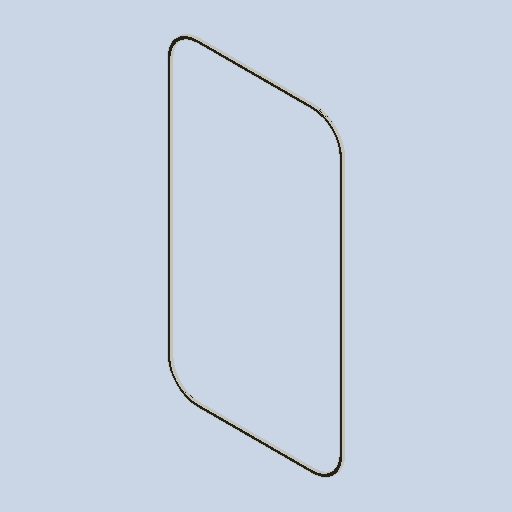
# Autodesk Inventor part: Caucho
Saved by Autodesk Inventor 2022.4 (Build 264492000, 492)
## iProperties
Created: 2022-11-28
Part Number: Caucho
Material: Generic
Document SubType Name: Sheet Metal
Designer: David
Density: 1 g/cm^3
Sheet Metal Rule: Default
Appearance: Gunmetal
Author: David
Autodesk Inventor part; units mm, degrees
ref_plane "YZ Plane" through (0, 0, 0) normal (1, 0, 0) x (0, 1, 0)
ref_plane "XZ Plane" through (0, 0, 0) normal (0, 1, 0) x (-1, 0, 0)
ref_plane "XY Plane" through (0, 0, 0) normal (0, 0, 1) x (1, 0, 0)
sketch "Sketch5" plane through (0, 0, 0) normal (0, 0, 1) x (1, 0, 0)
  line L0 (-300, -1100) -> (900, -1100)
  line L1 (900, -1100) -> (900, 850)
  line L2 (900, 850) -> (-300, 850)
  line L3 (-300, 850) -> (-300, -1100)
  line L4 (-300, -1100) -> (900, 850) construction
  line L5 (900, -1100) -> (-300, 850) construction
  line L6 (0, 700) -> (600, 700)
  line L7 (750, 550) -> (750, -800)
  line L8 (600, -950) -> (0, -950)
  line L9 (-150, -800) -> (-150, 550)
  arc A0 (750, 550) -> (600, 700) centre (600, 550) ccw
  arc A1 (0, 700) -> (-150, 550) centre (0, 550) ccw
  arc A2 (-150, -800) -> (0, -950) centre (0, -800) ccw
  arc A3 (600, -950) -> (750, -800) centre (600, -800) ccw
  line L10 (600, 697) -> (0, 697)
  arc A4 (0, 697) -> (-147, 550) centre (0, 550) ccw
  line L11 (-147, 550) -> (-147, -800)
  arc A5 (-147, -800) -> (0, -947) centre (0, -800) ccw
  line L12 (0, -947) -> (600, -947)
  arc A6 (600, -947) -> (747, -800) centre (600, -800) ccw
  line L13 (747, -800) -> (747, 550)
  arc A7 (747, 550) -> (600, 697) centre (600, 550) ccw
  point P0 (0, 0)
  point P1 (300, -125)
  dimension "d0" = 1200
  dimension "d1" = 1950
  dimension "d2" = 150
  dimension "d3" = 150
  dimension "d4" = 150
  dimension "d5" = 150
  dimension "d6" = 150
  dimension "d9" = 3
  constraints: 28 end point, 16 point on circle, 8 centre point, 8 tangent, 6 parallel, 3 perpendicular, 2 midpoint, 1 horizontal, 10 other
  measures "d0" distance of L2.end L1.end
  measures "d1" distance of L1.end L0.end
  measures "d2" distance between parallel lines of L2 L6
  measures "d3" radius of A0
  measures "d4" radius of A1
  measures "d5" radius of A2
  measures "d6" radius of A3
  measures "d9" distance between parallel lines of L6 L10
extrude "Extrusion1" add sketch "Sketch5" along normal mid plane 3.048 contours L6 A0 L7 A3 L8 A2 L9 A1
sketch "Sketch6" plane through (0, 0, 1.524) normal (0, 0, 1) x (1, 0, 0)
  line L0 (0, -950) -> (600, -950) projected
  arc A0 (600, -950) -> (750, -800) centre (600, -800) ccw projected
  line L1 (750, -800) -> (750, 550) projected
  arc A1 (750, 550) -> (600, 700) centre (600, 550) ccw projected
  line L2 (600, 700) -> (0, 700) projected
  arc A2 (0, 700) -> (-150, 550) centre (0, 550) ccw projected
  line L3 (-150, 550) -> (-150, -800) projected
  arc A3 (-150, -800) -> (0, -950) centre (0, -800) ccw projected
  arc A4 (747, 550) -> (600, 697) centre (600, 550) ccw projected
  line L4 (747, 550) -> (747, -800) projected
  arc A5 (600, -947) -> (747, -800) centre (600, -800) ccw projected
  line L5 (600, -947) -> (0, -947) projected
  arc A6 (-147, -800) -> (0, -947) centre (0, -800) ccw projected
  line L6 (-147, -800) -> (-147, 550) projected
  arc A7 (0, 697) -> (-147, 550) centre (0, 550) ccw projected
  line L7 (0, 697) -> (600, 697) projected
  line L8 (0, 708) -> (600, 708)
  arc A8 (758, 550) -> (600, 708) centre (600, 550) ccw
  line L9 (758, 550) -> (758, -800)
  arc A9 (600, -958) -> (758, -800) centre (600, -800) ccw
  line L10 (600, -958) -> (0, -958)
  arc A10 (-158, -800) -> (0, -958) centre (0, -800) ccw
  line L11 (-158, -800) -> (-158, 550)
  arc A11 (0, 708) -> (-158, 550) centre (0, 550) ccw
  arc A12 (741, 550) -> (600, 691) centre (600, 550) ccw
  line L12 (741, 550) -> (741, -800)
  arc A13 (600, -941) -> (741, -800) centre (600, -800) ccw
  line L13 (600, -941) -> (0, -941)
  arc A14 (-141, -800) -> (0, -941) centre (0, -800) ccw
  line L14 (-141, -800) -> (-141, 550)
  arc A15 (0, 691) -> (-141, 550) centre (0, 550) ccw
  line L15 (0, 691) -> (600, 691)
  point P0 (0, 0)
  dimension "d12" = 8
  dimension "d13" = 6
  constraints: 16 end point, 16 point on circle, 8 centre point, 14 other
  measures "d12" distance between parallel lines of L2 L8
  measures "d13" distance between parallel lines of L7 L15
extrude "Extrusion2" add sketch "Sketch6" along normal blind 4 contours A3 L3 A2 L2 A1 L1 A0 L0 | L4 A5 L5 A6 L6 A7 L7 A4 | L8 A8 L9 A9 L10 A10 L11 A11
sketch "Sketch7" plane through (0, 0, -1.524) normal (0, 0, -1) x (-1, 0, 0)
  line L0 (0, -958) -> (-600, -958) projected
  arc A0 (0, -958) -> (158, -800) centre (0, -800) ccw projected
  line L1 (158, 550) -> (158, -800) projected
  arc A1 (158, 550) -> (0, 708) centre (0, 550) ccw projected
  line L2 (-600, 708) -> (0, 708) projected
  arc A2 (-600, 708) -> (-758, 550) centre (-600, 550) ccw projected
  line L3 (-758, -800) -> (-758, 550) projected
  arc A3 (-758, -800) -> (-600, -958) centre (-600, -800) ccw projected
  arc A4 (0, -950) -> (150, -800) centre (0, -800) ccw projected
  line L4 (0, -950) -> (-600, -950) projected
  arc A5 (-750, -800) -> (-600, -950) centre (-600, -800) ccw projected
  line L5 (-750, -800) -> (-750, 550) projected
  arc A6 (-600, 700) -> (-750, 550) centre (-600, 550) ccw projected
  line L6 (-600, 700) -> (0, 700) projected
  arc A7 (150, 550) -> (0, 700) centre (0, 550) ccw projected
  line L7 (150, 550) -> (150, -800) projected
  line L8 (-600, -950) -> (0, -950) projected
  arc A8 (0, -950) -> (150, -800) centre (0, -800) ccw projected
  line L9 (150, -800) -> (150, 550) projected
  arc A9 (150, 550) -> (0, 700) centre (0, 550) ccw projected
  line L10 (0, 700) -> (-600, 700) projected
  arc A10 (-600, 700) -> (-750, 550) centre (-600, 550) ccw projected
  line L11 (-750, 550) -> (-750, -800) projected
  arc A11 (-750, -800) -> (-600, -950) centre (-600, -800) ccw projected
  arc A12 (-600, 697) -> (-747, 550) centre (-600, 550) ccw projected
  line L12 (-600, 697) -> (0, 697) projected
  arc A13 (147, 550) -> (0, 697) centre (0, 550) ccw projected
  line L13 (147, 550) -> (147, -800) projected
  arc A14 (0, -947) -> (147, -800) centre (0, -800) ccw projected
  line L14 (0, -947) -> (-600, -947) projected
  arc A15 (-747, -800) -> (-600, -947) centre (-600, -800) ccw projected
  line L15 (-747, -800) -> (-747, 550) projected
  line L16 (-600, -941) -> (0, -941) projected
  arc A16 (-741, -800) -> (-600, -941) centre (-600, -800) ccw projected
  line L17 (-741, 550) -> (-741, -800) projected
  arc A17 (-600, 691) -> (-741, 550) centre (-600, 550) ccw projected
  line L18 (0, 691) -> (-600, 691) projected
  arc A18 (141, 550) -> (0, 691) centre (0, 550) ccw projected
  line L19 (141, -800) -> (141, 550) projected
  arc A19 (0, -941) -> (141, -800) centre (0, -800) ccw projected
  line L20 (0, 697) -> (-600, 697) projected
  arc A20 (-600, 697) -> (-747, 550) centre (-600, 550) ccw projected
  line L21 (-747, 550) -> (-747, -800) projected
  arc A21 (-747, -800) -> (-600, -947) centre (-600, -800) ccw projected
  line L22 (-600, -947) -> (0, -947) projected
  arc A22 (0, -947) -> (147, -800) centre (0, -800) ccw projected
  line L23 (147, -800) -> (147, 550) projected
  arc A23 (147, 550) -> (0, 697) centre (0, 550) ccw projected
  point P0 (0, 0)
extrude "Extrusion3" add sketch "Sketch7" along normal blind 4 contours L0 A3 L3 A2 L2 A1 L1 A0 | L4 A5 L5 A6 L6 A7 L7 A4 | L12 A13 L13 A14 L14 A15 L15 A12
equation "\"d10\" = Thickness"
equation "\"BendRadius\" = Thickness"
equation "\"BendReliefWidth\" = Thickness"
equation "\"BendReliefDepth\" = 0.5 * Thickness"
equation "\"CornerReliefSize\" = 4 * Thickness"
equation "\"MinimumRemnant\" = 2 * Thickness"
equation "\"TransitionRadius\" = BendRadius"
equation "\"JacobiRadiusSize\" = BendRadius"
equation "\"GapSize\" = Thickness"
equation "\"Space7\" = 0"
equation "\"Thickness\" = 3.048"
body "Solid1"
